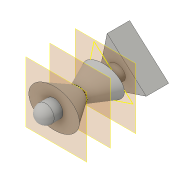
# Autodesk Inventor part: girlNT
Saved by Autodesk Inventor 2016 (Build 200138000, 138)
## iProperties
Created: 2016-01-28
Part Number: girlNT
Material: Generic
Document SubType Name: Modeling
Designer: 301278
Density: 1 g/cm^3
Appearance: Default
Author: 301278
Autodesk Inventor part; units mm, degrees
ref_plane "YZ Plane" through (0, 0, 0) normal (1, 0, 0) x (0, 1, 0)
ref_plane "XZ Plane" through (0, 0, 0) normal (0, 1, 0) x (-1, 0, 0)
ref_plane "XY Plane" through (0, 0, 0) normal (0, 0, 1) x (1, 0, 0)
sketch "Sketch1" plane through (0, 0, 0) normal (0, 0, 1) x (1, 0, 0)
  line L0 (-3.4267, 10.372) -> (10.6957, -2.2184)
  line L1 (10.6957, -2.2184) -> (-7.2691, -8.1536)
  line L2 (-7.2691, -8.1536) -> (-3.4267, 10.372)
  ellipse E0 centre (0, 0) end of major axis (3.175, 0) minor radius 2.667
  dimension "d1" = 3.175
  dimension "d2" = 2.667
  dimension "d0" = 14.1224
  constraints: 6 end point, 2 coincident, 9 other
  measures "d0" horizontal distance of L0.end L0.start
extrude "Extrusion1" add sketch "Sketch1" along normal blind 8.128 contours L0 L1 L2 | E0
ref_plane "Work Plane2" through (0, 0, 12.954) normal (0, 0, 1) x (1, 0, 0)
sketch "Sketch2" plane through (0, 0, 12.954) normal (0, 0, 1) x (1, 0, 0)
  point P0 (0, 0)
sketch "Sketch3" plane through (0, 0, 12.954) normal (0, 0, 1) x (1, 0, 0)
  point P0 (0, 0)
sketch "Sketch4" plane through (0, 0, 12.954) normal (0, 0, 1) x (1, 0, 0)
  ellipse E0 centre (0, 0) end of major axis (3.175, 0) minor radius 2.667
  dimension "d6" = 3.175
  dimension "d7" = 2.667
  constraints: 1 coincident, 2 other
sketch "Sketch5" plane through (0, 0, 12.954) normal (0, 0, 1) x (1, 0, 0)
  line L0 (10.6957, -2.2184) -> (-3.4267, 10.372) projected
  line L1 (-3.4267, 10.372) -> (-7.2691, -8.1536) projected
  line L2 (-7.2691, -8.1536) -> (10.6957, -2.2184) projected
sketch "Sketch6" plane through (0, 0, 8.128) normal (0, 0, 1) x (1, 0, 0)
  ellipse E0 centre (0, 0) end of major axis (3.175, 0) minor radius 2.667 projected
  ellipse E1 centre (0, 0) end of major axis (3.175, 0) minor radius 2.667
  constraints: 3 other
loft "Loft1" add profiles "Sketch6", "Sketch4"
ref_plane "Work Plane4" through (0, 0, 30.734) normal (0, 0, 1) x (1, 0, 0)
ref_plane "Work Plane3" through (0, 0, 22.098) normal (0, 0, 1) x (1, 0, 0)
sketch "Sketch7" plane through (0, 0, 22.098) normal (0, 0, 1) x (1, 0, 0)
  ellipse E0 centre (0, 0) end of major axis (-3.175, 0) minor radius 2.667 projected
  constraints: 1 other
sketch "Sketch8" plane through (0, 0, 22.098) normal (0, 0, 1) x (1, 0, 0)
  ellipse E0 centre (0, 0) end of major axis (3.175, 0) minor radius 2.667
  ellipse E1 centre (0, 0) end of major axis (-3.175, 0) minor radius 2.667 projected
  constraints: 1 coincident, 3 other
sketch "Sketch9" plane through (0, 0, 12.954) normal (0, 0, 1) x (1, 0, 0)
  ellipse E0 centre (0, 0) end of major axis (7.62, 0) minor radius 5.08
  dimension "d16" = 7.62
  dimension "d17" = 5.08
  constraints: 1 coincident, 2 other
loft "Loft2" add profiles "Sketch9", "Sketch7"
sketch "Sketch10" plane through (0, 0, 30.734) normal (0, 0, 1) x (1, 0, 0)
  ellipse E0 centre (0, 0) end of major axis (9.144, 0) minor radius 6.858
  dimension "d22" = 6.858
  dimension "d23" = 9.144
  constraints: 1 coincident, 2 other
loft "Loft3" add profiles "Sketch10" section 1 edges at (0, 2.667, 22.098) (0, -2.667, 22.098)
sketch "Sketch11" plane through (0, 0, 30.734) normal (0, 0, 1) x (1, 0, 0)
  line L0 (-3.175, 3.175) -> (3.175, 3.175)
  line L1 (3.175, 3.175) -> (3.175, -3.175)
  line L2 (3.175, -3.175) -> (-3.175, -3.175)
  line L3 (-3.175, -3.175) -> (-3.175, 3.175)
  point P0 (0, 0)
  dimension "d28" = 6.35
  dimension "d29" = 6.35
  dimension "d30" = 3.175
  dimension "d31" = 3.175
  constraints: 8 end point, 2 parallel, 1 horizontal, 1 perpendicular
  measures "d28" distance of L2.end L0.start
  measures "d29" distance of L0.end L0.start
  measures "d30" distance from line of point (0, 0) L1
  measures "d31" distance from line of L2 point (0, 0)
extrude "Extrusion2" add sketch "Sketch11" along normal blind 6.35
fillet "Fillet1" radius 3.175 1 edges at (3.175, 0, 37.084)
fillet "Fillet2" radius 3.175 1 edges at (-3.175, 0, 37.084)
fillet "Fillet3" radius 3.175 3 edges at (3.175, 3.175, 32.3215) (2.2451, 3.175, 36.1541) (-3.175, 3.175, 32.3215)
fillet "Fillet4" radius 3.175 3 edges at (3.175, -3.175, 32.3215) (2.2451, -3.175, 36.1541) (-3.175, -3.175, 32.3215)
body "Solid1"
